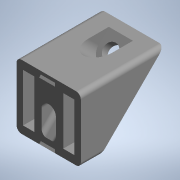
# Autodesk Inventor part: 14118
Saved by Autodesk Inventor 2021 (Build 250183000, 183)
## iProperties
Part Number: 14118
Material: Generic
Catalog Web Link: www.cadenas.de
Description: 14118-45 Deg. Support Connector
Vendor: 8020
Document SubType Name: Modeling
Designer: partserver
Manufacturer: 8020
Mass: 32.1586 g
Surface Area: 143.122 cm^2
Volume: 32.1586 cm^3
Density: 1 g/cm^3
Appearance: PSOLRGB-175-175-175
Category: PARTsolutions
Company: 8020
PSOL_IDENT_0: {$CADENAS_DATA\23d-libs\8020\metric\joining_plates\14118.prj},149 {VTYP=3D},{NB=14118},{LINA=14118},
PSOL_IDENT_1: {NN=14118},{DATE=31.07.2020 09:21:28},{GEOMDATE=27.02.2012 07:43:00},{VERSION=},{LINEID=10},{WBVAR=}
PSOL_IDENT_2: ,{WBNUMERIC=}  {NB=14118},{LINA=14118},{KT=DUMMY},{PN=14118},{MAT=Die-Cast Zinc},{FIN=Powder Coat Al
PSOL_IDENT_3: uminum Color},{A=52.00},{B=40.00},{C=9.00},{D=9.00},{E=9.00},{F=8.00},{G=45},{H=12.00},{J=3.20},{K=6
PSOL_IDENT_4: .000},{W=.214},{CC=8-40},{R1=3.000},{R2=3.500},{R3=15.500},{F1=15.000},{F2=7.500},{A1=10.000},{A2=12
PSOL_IDENT_5: .500},{A3=5.61593796},{A4=2.800},{A5=10.330},{A6=30.10050506},{A7=5.000}
NB: 14118
NN: 14118
NT: 45 Deg. Support Connector
NBSYN: $PN.
LINA: 14118
CATALOG: 80/20
PN: 14118
MAT: Die-Cast Zinc
FIN: Powder Coat Aluminum Color
A: 52
B: 40
C: 9
D: 9
E: 9
F: 8
G: 45
W: .214
CC: 8-40
SUPPLIER: 8020
ARTICLENO: 14118
BOMINFO: 14118
CREATOR: CADENAS GmbH
Title: 14118
Author: Cadenas PARTsolutions
Comments: 45 Deg. Support Connector
Autodesk Inventor part; units mm, degrees
ref_plane "YZ Plane" through (0, 0, 0) normal (1, 0, 0) x (0, 1, 0)
ref_plane "XZ Plane" through (0, 0, 0) normal (0, 1, 0) x (-1, 0, 0)
ref_plane "XY Plane" through (0, 0, 0) normal (0, 0, 1) x (1, 0, 0)
sketch "Sketch_1" plane through (0, 0, 0) normal (0, 1, 0) x (-1, 0, 0)
  arc A0 (20, 17) -> (17, 20) centre (17, 17) ccw
  line L0 (17, 20) -> (-17, 20)
  arc A1 (-17, 20) -> (-20, 17) centre (-17, 17) ccw
  line L1 (-20, 17) -> (-20, -17)
  arc A2 (-20, -17) -> (-17, -20) centre (-17, -17) ccw
  line L2 (-17, -20) -> (17, -20)
  arc A3 (17, -20) -> (20, -17) centre (17, -17) ccw
  line L3 (20, -17) -> (20, 17)
  constraints: 8 end point, 8 point on circle, 4 centre point
extrude "Extrusion1" add sketch "Sketch_1" along normal blind 52
sketch "Sketch_2" plane through (0, 0, 0) normal (1, 0, 0) x (0, 1, 0)
  line L0 (12, 20) -> (52, -20)
  line L1 (52, -20) -> (52, 20)
  line L2 (52, 20) -> (12, 20)
  constraints: 6 end point
extrude "Extrusion2" cut sketch "Sketch_2" along normal mid plane 40
sketch "Sketch_13" plane through (0, 0, 0) normal (1, 0, 0) x (0, 1, 0)
  line L0 (13.4142, 21.4142) -> (12, 20)
  line L1 (12, 20) -> (17.3033, 14.6967)
  line L2 (17.3033, 14.6967) -> (18.7175, 16.1109)
  line L3 (18.7175, 16.1109) -> (13.4142, 21.4142)
  constraints: 8 end point
extrude "Extrusion3" add sketch "Sketch_13" along normal mid plane 7.7
sketch "Sketch_14" plane through (0, 0, 0) normal (1, 0, 0) x (0, 1, 0)
  line L0 (47.7574, -12.9289) -> (46.3431, -14.3431)
  line L1 (46.3431, -14.3431) -> (52, -20)
  line L2 (52, -20) -> (53.4142, -18.5858)
  line L3 (53.4142, -18.5858) -> (47.7574, -12.9289)
  constraints: 8 end point
extrude "Extrusion4" add sketch "Sketch_14" along normal mid plane 7.7
sketch "Sketch_3" plane through (0, 15.5, 0) normal (0, 1, 0) x (1, 0, 0)
  line L0 (-16.8, -23.5) -> (-10.8, -23.5)
  line L1 (-10.8, -23.5) -> (-10.8, 16.5)
  line L2 (-10.8, 16.5) -> (-16.8, 16.5)
  line L3 (-16.8, 16.5) -> (-16.8, -23.5)
  constraints: 8 end point
extrude "Extrusion5" cut sketch "Sketch_3" along normal blind 40
sketch "Sketch_4" plane through (0, 15.5, 0) normal (0, 1, 0) x (1, 0, 0)
  line L0 (10.8, -23.5) -> (16.8, -23.5)
  line L1 (16.8, -23.5) -> (16.8, 16.5)
  line L2 (16.8, 16.5) -> (10.8, 16.5)
  line L3 (10.8, 16.5) -> (10.8, -23.5)
  constraints: 8 end point
extrude "Extrusion6" cut sketch "Sketch_4" along normal blind 40
sketch "Sketch_5" plane through (0, 10, 0) normal (0, 1, 0) x (1, 0, 0)
  line L0 (-7.5, 0.5) -> (-7.5, -7.5)
  line L1 (-7.5, -7.5) -> (7.5, -7.5)
  line L2 (7.5, -7.5) -> (7.5, 0.5)
  arc A0 (7.5, 0.5) -> (-7.5, 0.5) centre (0, 0.5) ccw
  constraints: 6 end point, 2 point on circle, 1 centre point
extrude "Extrusion7" cut sketch "Sketch_5" along normal blind 40
sketch "Sketch_6" plane through (0, 0, 0) normal (1, 0, 0) x (0, 1, 0)
  line L0 (50, 20) -> (22.5, 20)
  line L1 (22.5, 20) -> (10, 7.5)
  line L2 (10, 7.5) -> (50, 7.5)
  line L3 (50, 7.5) -> (50, 20)
  constraints: 8 end point
extrude "Extrusion8" cut sketch "Sketch_6" along normal mid plane 15
sketch "Sketch9" plane through (0, 10, 0) normal (0, 1, 0) x (1, 0, 0)
  point P0 (0, 0)
hole "Hole1" at (0, 10, 0) direction (0, -1, 0) diameter 9 depth 10
sketch "Sketch_8" plane through (0, 0, 14.3841) normal (0, -0.7071, 0.7071) x (1, 0, 0)
  line L0 (-4.5, -2.7) -> (-4.5, -3.5714)
  line L1 (-4.5, -3.5714) -> (4.5, -3.5714)
  line L2 (4.5, -3.5714) -> (4.5, -2.7)
  arc A0 (4.5, -2.7) -> (1.8, 0) centre (1.8, -2.7) ccw
  line L3 (1.8, 0) -> (-1.8, 0)
  arc A1 (-1.8, 0) -> (-4.5, -2.7) centre (-1.8, -2.7) ccw
  constraints: 8 end point, 4 point on circle, 2 centre point
extrude "Extrusion9" cut sketch "Sketch_8" against normal blind 20
sketch "Sketch_9" plane through (0, 0, 0) normal (1, 0, 0) x (0, 1, 0)
  line L0 (0, 9.67) -> (0, 0)
  line L1 (0, 0) -> (10, 0)
  line L2 (10, 0) -> (10, 4.3841)
  line L3 (10, 4.3841) -> (4.7141, 9.67)
  line L4 (4.7141, 9.67) -> (0, 9.67)
  constraints: 10 end point
extrude "Extrusion10" cut sketch "Sketch_9" along normal mid plane 3
sketch "Sketch_10" plane through (0, 0, 0) normal (1, 0, 0) x (0, 1, 0)
  line L0 (0.7957, 9.77) -> (0, 9.77)
  line L1 (0, 9.77) -> (0, 0)
  line L2 (0, 0) -> (10, 0)
  line L3 (10, 0) -> (10, 0.5657)
  line L4 (10, 0.5657) -> (0.7957, 9.77)
  constraints: 10 end point
extrude "Extrusion11" cut sketch "Sketch_10" along normal mid plane 9
sketch "Sketch_11" plane through (0, 0, 0) normal (1, 0, 0) x (0, 1, 0)
  line L0 (27.9584, -24.2426) -> (42.1005, -10.1005)
  line L1 (42.1005, -10.1005) -> (45.2825, -13.2825)
  line L2 (45.2825, -13.2825) -> (31.1403, -27.4246)
  line L3 (31.1403, -27.4246) -> (27.9584, -24.2426)
  line L4 (27.9584, -24.2426) -> (42.1005, -10.1005)
  constraints: 10 end point
revolve "Revolution1" cut sketch "Sketch_11" angle 360 about axis through (0, 27.9584, -24.2426) along (0, -0.7071, -0.7071)
sketch "Sketch_15" plane through (0, 0, 0) normal (1, 0, 0) x (0, 1, 0)
  line L0 (0, 20) -> (-2, 18)
  line L1 (-2, 18) -> (-0.9393, 16.9393)
  line L2 (-0.9393, 16.9393) -> (1.0607, 18.9393)
  line L3 (1.0607, 18.9393) -> (0, 20)
  constraints: 8 end point
extrude "Extrusion12" add sketch "Sketch_15" along normal mid plane 8
sketch "Sketch_16" plane through (0, 0, 0) normal (1, 0, 0) x (0, 1, 0)
  line L0 (0, -15.8787) -> (-2, -17.8787)
  line L1 (-2, -17.8787) -> (-0.9393, -18.9393)
  line L2 (-0.9393, -18.9393) -> (1.0607, -16.9393)
  line L3 (1.0607, -16.9393) -> (0, -15.8787)
  constraints: 8 end point
extrude "Extrusion13" add sketch "Sketch_16" along normal mid plane 8
sketch "Sketch_12" plane through (0, 28.4645, -3.5355) normal (0, 0.7071, 0.7071) x (1, 0, 0)
  arc A0 (-7.5, 14.3) -> (7.5, 14.3) centre (0, 14.3) ccw
  line L0 (7.5, 14.3) -> (7.5, 23.3)
  line L1 (7.5, 23.3) -> (-7.5, 23.3)
  line L2 (-7.5, 23.3) -> (-7.5, 14.3)
  constraints: 6 end point, 2 point on circle, 1 centre point
extrude "Extrusion14" cut sketch "Sketch_12" against normal blind 40
sketch "Sketch_17" plane through (9, 0, 0) normal (1, 0, 0) x (0, 0, -1)
  line L0 (-15, 12.5) -> (-15, 0)
  line L1 (-15, 0) -> (15, 0)
  line L2 (15, 0) -> (2.5, 12.5)
  line L3 (2.5, 12.5) -> (-15, 12.5)
  constraints: 8 end point
extrude "Extrusion15" cut sketch "Sketch_17" along normal blind 7
sketch "Sketch_18" plane through (-9, 0, 0) normal (1, 0, 0) x (0, 0, -1)
  line L0 (-15, 12.5) -> (-15, 0)
  line L1 (-15, 0) -> (15, 0)
  line L2 (15, 0) -> (2.5, 12.5)
  line L3 (2.5, 12.5) -> (-15, 12.5)
  constraints: 8 end point
extrude "Extrusion16" cut sketch "Sketch_18" against normal blind 7
body "Solid1"
